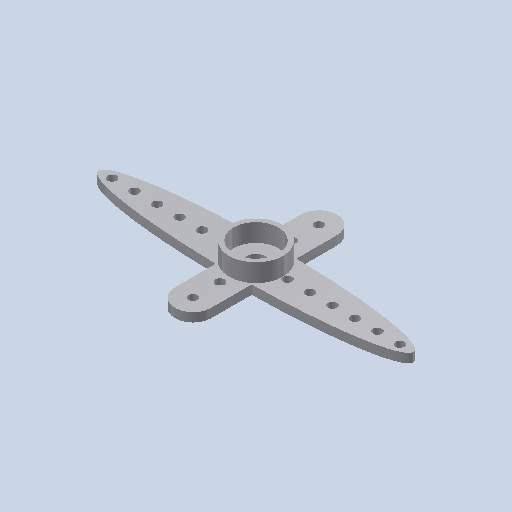
# Autodesk Inventor part: Part1
Saved by Autodesk Inventor 2024 (Build 280153000, 153)
## iProperties
Created: 2017-05-25
Part Number: Part1
Material: PVC-Piping
Document SubType Name: Modeling
Designer: L.Đ.P
Density: 1.4 g/cm^3
Appearance: Smooth - White
Author: L.Đ.P
Autodesk Inventor part; units mm, degrees
ref_plane "YZ Plane" through (0, 0, 0) normal (1, 0, 0) x (0, 1, 0)
ref_plane "XZ Plane" through (0, 0, 0) normal (0, 1, 0) x (-1, 0, 0)
ref_plane "XY Plane" through (0, 0, 0) normal (0, 0, 1) x (1, 0, 0)
sketch "Sketch1" plane through (0, 0, 0) normal (0, 0, 1) x (1, 0, 0)
  ellipse E0 centre (0, 0) end of major axis (-17.5, 0) minor radius 2.5
  line L0 (0, 0) -> (0, -2.5)
  dimension "d0" = 17.5
  dimension "d1" = 2.5
  constraints: 2 end point, 1 coincident, 1 vertical, 1 vertical alignment, 2 other
  measures "d1" distance of L0.start L0.end
extrude "Extrusion1" add sketch "Sketch1" along normal mid plane 1
sketch "Sketch2" plane through (0, 0, 0.5) normal (0, 0, 1) x (1, 0, 0)
  ellipse E0 centre (0, 0) end of major axis (17.5, 0) minor radius 2.5 projected
  circle A0 centre (0, 0) radius 3
  dimension "d4" = 6
  constraints: 1 centre point, 1 coincident, 1 other
  measures "d4" diameter of A0
extrude "Extrusion2" add sketch "Sketch2" along normal blind 2 and the other way blind 1 contours A0 E0 | E0 A0 | A0 E0 picked at (1.5591, 0) picked at (0.3978, 2.6587) picked at (0.3978, -2.6587)
sketch "Sketch3" plane through (0, 0, 2.5) normal (0, 0, 1) x (1, 0, 0)
  circle A0 centre (0, 0) radius 3 projected
  circle A1 centre (0, 0) radius 2.5
  dimension "d7" = 5
  constraints: 1 centre point, 1 coincident
  measures "d7" diameter of A1
extrude "Extrusion3" cut sketch "Sketch3" against normal blind 2 contours A1
sketch "Sketch4" plane through (0, 0, -0.5) normal (0, 0, -1) x (-1, 0, 0)
  ellipse E0 centre (0, 0) end of major axis (-17.5, 0) minor radius 2.5 projected
  circle A0 centre (0, 0) radius 2
  dimension "d10" = 4
  constraints: 1 centre point, 1 coincident, 1 other
  measures "d10" diameter of A0
extrude "Extrusion4" cut sketch "Sketch4" against normal blind 0.5 contours A0
sketch "Sketch5" plane through (0, 0, 0) normal (0, 0, -1) x (-1, 0, 0)
  circle A0 centre (0, 0) radius 2 projected
  circle A1 centre (0, 0) radius 1
  dimension "d13" = 2
  constraints: 1 centre point, 1 coincident
  measures "d13" diameter of A1
extrude "Extrusion5" cut sketch "Sketch5" against normal through all contours A1
sketch "Sketch6" plane through (0, 0, -0.5) normal (0, 0, -1) x (-1, 0, 0)
  ellipse E0 centre (0, 0) end of major axis (-17.5, 0) minor radius 2.5 projected
  circle A0 centre (-16, 0) radius 0.5
  line L0 (0, 0) -> (0, -1.2687)
  line L1 (0, 0) -> (-1.4808, 0)
  dimension "d16" = 1
  dimension "d17" = 16
  constraints: 4 end point, 1 centre point, 1 perpendicular, 1 point on line, 1 vertical, 1 other
  measures "d16" diameter of A0
  measures "d17" distance of L0.start A0.centre
extrude "Extrusion6" cut sketch "Sketch6" against normal through all contours A0
pattern_linear "Rectangular Pattern1" count 6 spacing 2.5 along (-1, 0, 0) of "Extrusion6"
mirror "Mirror2" about plane through (0, 0, 0) normal (1, 0, 0) of "Extrusion6", "Rectangular Pattern1"
sketch "Sketch7" plane through (0, 0, -0.5) normal (0, 0, -1) x (-1, 0, 0)
  circle A0 centre (0, 0) radius 2 projected
  arc A1 (1.6755, 2.4885) -> (-1.6755, 2.4885) centre (0, 0) ccw projected
  line L0 (2, -7) -> (-2, -7)
  line L1 (-2, -7) -> (-2, 7)
  line L2 (-2, 7) -> (2, 7)
  line L3 (2, 7) -> (2, -7)
  line L4 (0, 0) -> (0, 1.4793)
  line L5 (0, 0) -> (-1.001, 0)
  circle A2 centre (0, 7) radius 2
  circle A3 centre (0, -7) radius 2
  circle A4 centre (0, 0) radius 2
  point P0 (2, 0)
  dimension "d25" = 4
  dimension "d26" = 14
  constraints: 12 end point, 3 midpoint, 3 parallel, 2 coincident, 2 horizontal alignment, 2 perpendicular, 2 point on line, 1 centre point, 1 concentric, 1 horizontal, 4 other
  measures "d25" distance of L1.end L2.end
  measures "d26" distance of L0.end L1.end
extrude "Extrusion7" add sketch "Sketch7" against normal blind 1 contours L3 A3 L1 A0 | A0 L1 A2 L3 | A2 L2 | L2 A2 | A3 L0 | L0 A3
sketch "Sketch8" plane through (0, 0, -0.5) normal (0, 0, -1) x (-1, 0, 0)
  arc A0 (2, 7) -> (-2, 7) centre (0, 7) ccw projected
  circle A1 centre (0, 7) radius 0.5
  dimension "d29" = 1
  constraints: 1 centre point, 1 coincident
  measures "d29" diameter of A1
extrude "Extrusion8" cut sketch "Sketch8" against normal blind 1
pattern_linear "Rectangular Pattern2" count 2 spacing 3 along (0, -1, 0) of "Extrusion8"
mirror "Mirror3" about plane through (0, 0, 0) normal (0, 1, 0) of "Extrusion8", "Rectangular Pattern2"
body "Solid1"
